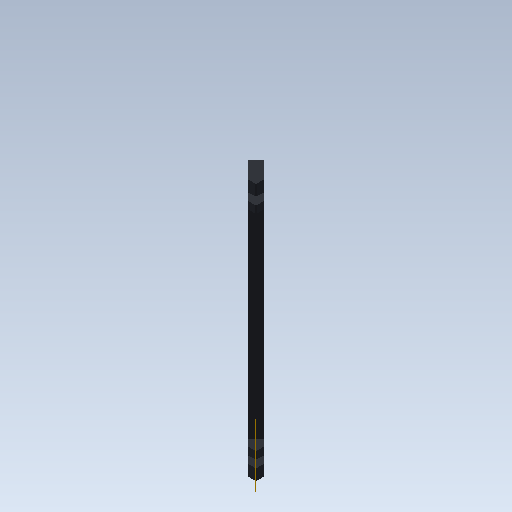
# Autodesk Inventor part: Standard
Saved by Autodesk Inventor 2020.3 (Build 243373000, 373)
## iProperties
RuleStatus: InUse
AfterDocSave0: file://Part Number Cleaner
Created: 2023-03-03
Material: ABS, BLACK
Catalog Web Link: https://www.janelia.org/
Vendor: HHMI: JRC - jET
Document SubType Name: Modeling
Designer: jalala
Density: 1.06 g/cm^3
Appearance: Black Anodize
DESIGN DEPARTMENT: HHMI: JRC - jET
ALTERED ITEM PART NUMBER: N/A
ALTERED ITEM VENDOR: N/A
ALTERED ITEM DESCRIPTION: N/A
Title: Standard
Author: jalala
Revision Number: 0
Autodesk Inventor part; units mm, degrees
ref_plane "YZ Plane" through (0, 0, 0) normal (1, 0, 0) x (0, 1, 0)
ref_plane "XZ Plane" through (0, 0, 0) normal (0, 1, 0) x (-1, 0, 0)
ref_plane "XY Plane" through (0, 0, 0) normal (0, 0, 1) x (1, 0, 0)
ref_plane "Work Plane1" through (29.21, 0, 29.21) normal (0.7071, 0, -0.7071) x (0, 1, 0)
sketch "Sketch1" plane through (29.21, 0, 29.21) normal (0.7071, 0, -0.7071) x (0, 1, 0)
  line L0 (0, -10.8661) -> (0, -7.5614) construction
  line L1 (-0.127, -8.4271) -> (-0.127, -2.0771)
  line L2 (-0.127, -2.0771) -> (-4.8895, -2.0771)
  line L3 (-4.8895, -2.0771) -> (-4.8895, -14.7771)
  line L4 (-0.127, -8.4271) -> (3.175, -8.4271)
  line L5 (3.175, -8.4271) -> (3.175, -2.0771)
  line L6 (3.175, -2.0771) -> (6.35, -2.0771)
  line L7 (6.35, -2.0771) -> (6.35, -8.4271)
  line L8 (6.35, -8.4271) -> (50.8, -8.4271)
  line L9 (3.175, -0.3592) -> (3.175, -41.4888) construction
  line L10 (0, -8.4271) -> (3.175, -8.4271) construction
  line L11 (-4.8895, -14.7771) -> (50.8, -14.7771)
  line L12 (50.8, -8.4271) -> (50.8, -26.7173) construction
  line L13 (101.6, -10.8661) -> (101.6, -7.5614) construction
  line L14 (101.727, -8.4271) -> (101.727, -2.0771)
  line L15 (101.727, -2.0771) -> (106.4895, -2.0771)
  line L16 (106.4895, -2.0771) -> (106.4895, -14.7771)
  line L17 (101.727, -8.4271) -> (98.425, -8.4271)
  line L18 (98.425, -8.4271) -> (98.425, -2.0771)
  line L19 (98.425, -2.0771) -> (95.25, -2.0771)
  line L20 (95.25, -2.0771) -> (95.25, -8.4271)
  line L21 (95.25, -8.4271) -> (50.8, -8.4271)
  line L22 (98.425, -0.3592) -> (98.425, -41.4888) construction
  line L23 (101.6, -8.4271) -> (98.425, -8.4271) construction
  line L24 (106.4895, -14.7771) -> (50.8, -14.7771)
  point P0 (0, -41.3092)
  dimension "d0" = 0.127
  dimension "d1" = 4.7625
  dimension "d2" = 12.7
  dimension "d3" = 3.175
  dimension "d4" = 6.35
  dimension "d5" = 6.35
  dimension "d6" = 47.625
  constraints: 46 end point, 14 symmetric about line, 8 point on line, 4 horizontal, 4 perpendicular, 2 vertical, 2 other
  measures "d0" distance between parallel lines of L0 L1
  measures "d1" distance of L1.end L2.end
  measures "d2" distance of L2.end L3.end
  measures "d3" distance of L5.end L6.end
  measures "d4" distance from line of L3.end L4
  measures "d5" distance between parallel lines of L8 L6
  measures "d6" distance from line of L8.end L5
extrude "Extrusion1" add sketch "Sketch1" along normal mid plane 5.08
sketch "Sketch2" plane through (20.557, -4.8895, 16.9649) normal (0, -1, 0) x (0.7071, 0, -0.7071)
  line L0 (-2.54, 14.4179) -> (38.5896, -26.7117) construction
  line L1 (-43.49, -26.5321) -> (-2.54, 14.4179) construction
  line L2 (-2.54, 12.9811) -> (1.3375, 9.1035)
  line L3 (-2.54, 12.9811) -> (-7.1002, 8.4208)
  line L4 (-7.1002, 8.4208) -> (-7.1002, 14.2653)
  line L5 (-7.1002, 14.2653) -> (1.3375, 14.2653)
  line L6 (1.3375, 14.2653) -> (1.3375, 9.1035)
  point P0 (-2.54, -26.5321)
  dimension "d9" = 1.016
  dimension "d10" = 1.016
  dimension "d11" = 8.4378
  dimension "d12" = 5.1618
  constraints: 10 end point, 2 perpendicular, 2 vertical
  measures "d9" distance between parallel lines of L1 L3
  measures "d10" distance between parallel lines of L0 L2
  measures "d11" distance of L4.end L5.end
  measures "d12" distance of L5.end L2.end
extrude "Extrusion2" cut sketch "Sketch2" against normal through all
body "Solid1"
